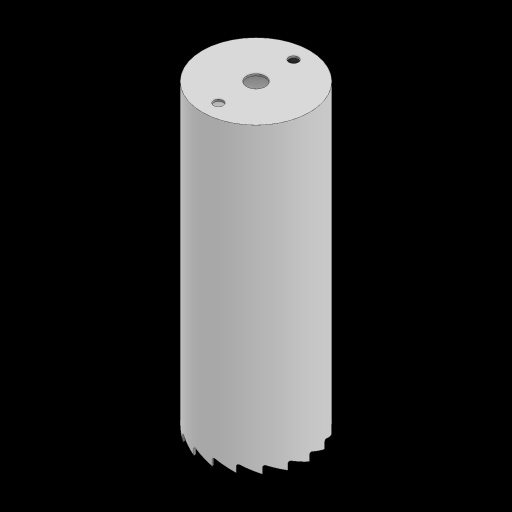
# Autodesk Inventor part: SC-1-01- Hole Saw
Saved by Autodesk Inventor 2023 (Build 270158000, 158)
## iProperties
Created: 2023-12-30
Part Number: SC-1-01- Hole Saw
Material: Generic
Document SubType Name: Modeling
Designer: annah
Density: 1 g/cm^3
Appearance: Default
Author: annah
Autodesk Inventor part; units mm, degrees
ref_plane "YZ Plane" through (0, 0, 0) normal (1, 0, 0) x (0, 1, 0)
ref_plane "XZ Plane" through (0, 0, 0) normal (0, 1, 0) x (-1, 0, 0)
sketch "Sketch1" plane through (0, 0, 0) normal (0, 1, 0) x (-1, 0, 0)
  circle A0 centre (0, 0) radius 17.4625
  circle A1 centre (0, 0) radius 18.0975
  dimension "d0" = 34.925
  dimension "d4" = 36.195
  constraints: 2 centre point, 2 coincident
  measures "d0" diameter of A0
  measures "d4" diameter of A1
extrude "Extrusion2" add sketch "Sketch1" against normal blind 101.6
extrude "Extrusion3" add sketch "Sketch1" along normal blind 0.635 contours A0 | A1
sketch "Sketch3" plane through (0, 0.635, 0) normal (0, 1, 0) x (1, 0, 0)
  circle A0 centre (0, 0) radius 3.175
  circle A1 centre (0, -12.7) radius 1.5875
  circle A2 centre (0, 12.7) radius 1.5875
  dimension "d9" = 6.35
  dimension "d45" = 3.175
  dimension "d46" = 3.175
  dimension "d47" = 12.7
  dimension "d48" = 12.7
  constraints: 3 centre point, 1 coincident
  measures "d9" diameter of A0
  measures "d45" diameter of A1
  measures "d46" diameter of A2
  measures "d47" distance of A2.centre point (0, 0)
  measures "d48" distance of A1.centre point (0, 0)
extrude "Extrusion4" cut sketch "Sketch3" against normal up to surface (0.635 mm away) contours A0
ref_plane "Work Plane1" through (0, 0, 18.0975) normal (0, 0, 1) x (1, 0, 0)
sketch "Sketch5" plane through (0, 0, 18.0975) normal (0, 0, 1) x (1, 0, 0)
  line L0 (-18.0975, -101.6) -> (18.0975, -101.6) projected
  line L1 (0, -101.6) -> (3.175, -101.6)
  line L2 (0, -101.6) -> (-3.175, -101.6)
  line L3 (-3.175, -101.6) -> (-3.175, -98.679)
  line L4 (-3.175, -98.679) -> (3.175, -101.6)
  point P0 (0, 0)
  dimension "d13" = 3.175
  dimension "d14" = 3.175
  dimension "d19" = 2.921
  constraints: 8 end point, 2 point on line, 1 midpoint, 1 perpendicular
  measures "d13" distance of L1.end L1.start
  measures "d14" distance of L2.end L1.start
  measures "d19" distance of L2.end L3.end
extrude "Extrusion5" cut sketch "Sketch5" against normal up to surface
pattern_circular "Circular Pattern1" count 18 over 360 about axis through (0, -10, 0) along (0, 1, 0) of "Extrusion5"
fillet "Face Fillet1" radius 0.5588 1 edges at (-3.175, -98.679, 17.4941)
pattern_circular "Circular Pattern2" count 18 over 360 about axis through (0, -10, 0) along (0, 1, 0) of "Face Fillet1"
extrude "Extrusion6" cut sketch "Sketch3" against normal up to surface (0.635 mm away) contours A1 | A2
equation "\"d48\" = d47"
equation "\"d14\" = d13"
body "Solid2"
